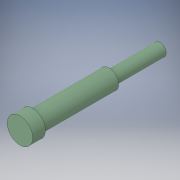
# Autodesk Inventor part: leg_1
Saved by Autodesk Inventor 2018 (Build 220112000, 112)
## iProperties
Created: 2018-10-25
Part Number: leg_1
Material: Generic
Document SubType Name: Modeling
Designer: iki
Density: 1 g/cm^3
Appearance: Default
Author: iki
Autodesk Inventor part; units mm, degrees
ref_plane "YZ Plane" through (0, 0, 0) normal (1, 0, 0) x (0, 1, 0)
ref_plane "XZ Plane" through (0, 0, 0) normal (0, 1, 0) x (-1, 0, 0)
ref_plane "XY Plane" through (0, 0, 0) normal (0, 0, 1) x (1, 0, 0)
sketch "Sketch1" plane through (0, 0, 0) normal (0, 1, 0) x (-1, 0, 0)
  circle A0 centre (0, 0) radius 5
  dimension "d0" = 10
  constraints: 1 centre point, 1 coincident
  measures "d0" diameter of A0
extrude "Extrusion1" add sketch "Sketch1" along normal blind 5
sketch "Sketch2" plane through (0, 5, 0) normal (0, 1, 0) x (1, 0, 0)
  circle A0 centre (0, 0) radius 3.75
  dimension "d3" = 7.5
  constraints: 1 centre point, 1 coincident
  measures "d3" diameter of A0
extrude "Extrusion2" add sketch "Sketch2" along normal blind 30
sketch "Sketch3" plane through (0, 35, 0) normal (0, 1, 0) x (1, 0, 0)
  circle A0 centre (0, 0) radius 2.45
  dimension "d6" = 4.9
  constraints: 1 centre point, 1 coincident
  measures "d6" diameter of A0
extrude "Extrusion3" add sketch "Sketch3" along normal blind 20
body "Solid1"
